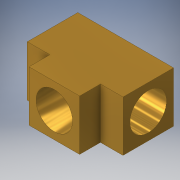
# Autodesk Inventor part: PPPP
Saved by Autodesk Inventor 2016 SP2 (Build 200236200, 236)
## iProperties
Created: 2017-03-28
Part Number: PPPP
Material: Brass
Document SubType Name: Modeling
Designer: smiku
Mass: 31.2871 g
Surface Area: 31.0439 cm^2
Volume: 3.68517 cm^3
Density: 8.49 g/cm^3
Appearance: Brass - Polished
Author: smiku
Autodesk Inventor part; units mm, degrees
note: some values were not read from the file. Chosen so that the rebuilt part matches the saved one: direction of "Hole2".
ref_plane "YZ Plane" through (0, 0, 0) normal (1, 0, 0) x (0, 1, 0)
ref_plane "XZ Plane" through (0, 0, 0) normal (0, 1, 0) x (-1, 0, 0)
ref_plane "XY Plane" through (0, 0, 0) normal (0, 0, 1) x (1, 0, 0)
sketch "Sketch1" plane through (0, 0, 0) normal (0, 0, 1) x (1, 0, 0)
  line L0 (-13.4747, -7.1247) -> (13.4747, -7.1247)
  line L1 (13.4747, -7.1247) -> (13.4747, 7.1247)
  line L2 (13.4747, 7.1247) -> (-13.4747, 7.1247)
  line L3 (-13.4747, 7.1247) -> (-13.4747, -7.1247)
  line L4 (-13.4747, -7.1247) -> (13.4747, 7.1247) construction
  line L5 (13.4747, -7.1247) -> (-13.4747, 7.1247) construction
  line L6 (-7.1247, -7.1247) -> (7.1247, -7.1247)
  line L7 (7.1247, -7.1247) -> (7.1247, 7.1247)
  line L8 (7.1247, 7.1247) -> (-7.1247, 7.1247)
  line L9 (-7.1247, 7.1247) -> (-7.1247, -7.1247)
  line L10 (-7.1247, -7.1247) -> (7.1247, 7.1247) construction
  line L11 (7.1247, -7.1247) -> (-7.1247, 7.1247) construction
  point P0 (0, 0)
  dimension "d0" = 26.9494
  dimension "d1" = 14.2494
  dimension "d2" = 14.2494
  constraints: 24 end point, 4 midpoint, 4 parallel, 2 horizontal, 2 perpendicular, 1 point on line
  measures "d0" distance of L2.end L1.end
  measures "d1" distance of L0.end L1.end
  measures "d2" distance of L8.end L7.end
extrude "Extrusion1" add sketch "Sketch1" along normal blind 5.8674 contours L9 L2 L7 L0
extrude "Extrusion2" add sketch "Sketch1" against normal blind 14.224
sketch "Sketch2" plane through (13.4747, -7.1247, 0) normal (1, 0, 0) x (0, 0, -1)
  line L0 (0, 0) -> (0, 14.2494) construction
  line L1 (0, 0) -> (14.224, 0) construction
  line L2 (14.224, 14.2494) -> (14.224, 0) construction
  line L3 (0, 14.2494) -> (14.224, 14.2494) construction
  circle A0 centre (7.0993, 7.1247) radius 7.1247 construction
  point P0 (0, 7.1247)
  constraints: 3 tangent, 1 centre point, 1 coincident
hole "Hole1" at (13.4747, 0, -7.0993) direction (-1, 0, 0) diameter 10.3124 end through all
sketch "Sketch3" plane through (0, 0, 5.8674) normal (0, 0, 1) x (1, 0, 0)
  point P0 (0, 0)
  point P1 (0, 0)
  constraints: 1 coincident
hole "Hole2" at (0, 0, 5.8674) direction (0, 0, -1) diameter 10.3124 end up to surface
body "Solid1"
